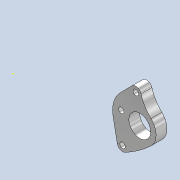
# Autodesk Inventor part: 前足フレーム補助パーツ
Saved by Autodesk Inventor 2020 (Build 240168000, 168)
## iProperties
Created: 2021-02-23
Part Number: 前足フレーム補助パーツ
Material: アルミニウム 2014-T6
Document SubType Name: Modeling
Designer: AA19065
Density: 2.78927 g/cm^3
Appearance: サテン
Mass: 6.98689 g
Surface Area: 17.7463 cm^2
Volume: 2.50492 cm^3
Author: AA19065
Autodesk Inventor part; units mm, degrees
ref_plane "YZ Plane" through (0, 0, 0) normal (1, 0, 0) x (0, 1, 0)
ref_plane "XZ Plane" through (0, 0, 0) normal (0, 1, 0) x (-1, 0, 0)
ref_plane "XY Plane" through (0, 0, 0) normal (0, 0, 1) x (1, 0, 0)
sketch "スケッチ1" plane through (0, 0, 0) normal (0, 0, 1) x (1, 0, 0)
  circle A0 centre (70, 10) radius 6.025
  circle A1 centre (70, 10) radius 9
  arc A2 (70.8604, 37.0956) -> (76.1852, 16.5379) centre (89.93, 31.0664) ccw
  arc A3 (-3.9904, -8.067) -> (76.0896, 3.373) centre (27.7113, 56.0206) ccw
  arc A4 (70.6777, 25.6489) -> (65.6559, 26.9449) centre (67.7899, 24.8363) ccw
  arc A5 (59.3301, 20.543) -> (55.2759, 7.1361) centre (70, 10) ccw
  arc A6 (57.575, -4.684) -> (61.9566, -6.7447) centre (60.5198, -4.1112) ccw
  line L0 (67.7899, 24.8363) -> (70, 10) construction
  line L1 (70, 10) -> (60.5198, -4.1112) construction
  circle A7 centre (67.7899, 24.8363) radius 1.5
  circle A8 centre (60.5198, -4.1112) radius 1.5
  line L2 (70, 10) -> (59.7573, 12.3103) construction
  circle A9 centre (59.7573, 12.3103) radius 1.5
  line L3 (59.3301, 20.543) -> (65.6559, 26.9449)
  line L4 (55.2759, 7.1361) -> (57.575, -4.684)
  point P0 (0, 0)
  point P1 (0, 0)
  dimension "d0" = 3
  dimension "d1" = 3
  dimension "d2" = 3
  dimension "d3" = 3
  dimension "d4" = 3
  dimension "d5" = 15
  dimension "d6" = 17
  constraints: 13 point on circle, 10 centre point, 10 end point, 7 tangent, 3 coincident, 1 concentric, 1 equal radius, 1 point on line, 9 other
  measures "d0" radius of A4
  measures "d1" diameter of A7
  measures "d2" diameter of A8
  measures "d3" diameter of A9
  measures "d5" distance of L0.start L0.end
  measures "d6" distance of L0.end L1.end
extrude "押し出し1" add sketch "スケッチ1" along normal blind 6
sketch "スケッチ2" plane through (0, 0, 6) normal (0, 0, 1) x (1, 0, 0)
  point P0 (0, 0)
sketch "スケッチ3" plane through (0, 0, 6) normal (0, 0, 1) x (1, 0, 0)
  line L0 (65.6559, 26.9449) -> (59.3301, 20.543) projected
  arc A0 (59.3301, 20.543) -> (55.2759, 7.1361) centre (70, 10) ccw projected
  line L1 (55.2759, 7.1361) -> (57.575, -4.684) projected
  arc A1 (57.575, -4.684) -> (61.9566, -6.7447) centre (60.5198, -4.1112) ccw projected
  arc A2 (61.9566, -6.7447) -> (76.0896, 3.373) centre (27.7113, 56.0206) ccw projected
  arc A3 (76.0896, 3.373) -> (76.1852, 16.5379) centre (70, 10) ccw projected
  arc A4 (70.6777, 25.6489) -> (76.1852, 16.5379) centre (89.93, 31.0664) ccw projected
  arc A5 (70.6777, 25.6489) -> (65.6559, 26.9449) centre (67.7899, 24.8363) ccw projected
  circle A6 centre (70, 10) radius 6.025 projected
  circle A7 centre (59.7573, 12.3103) radius 1.5 projected
  circle A8 centre (67.7899, 24.8363) radius 1.5 projected
  circle A9 centre (60.5198, -4.1112) radius 1.5 projected
  circle A10 centre (70, 10) radius 8
  line L2 (65.9307, 16.8878) -> (72.7106, 20.8933)
  line L3 (63.4649, 5.3856) -> (68.9527, -2.3863)
  point P0 (0, 0)
  dimension "d9" = 16
  constraints: 4 end point, 4 point on circle, 2 line through centre, 2 tangent, 1 centre point, 1 coincident
  measures "d9" diameter of A10
extrude "押し出し2" cut sketch "スケッチ3" against normal blind 3 contours A4 A3 A2 L3 A10 L2 | A10
